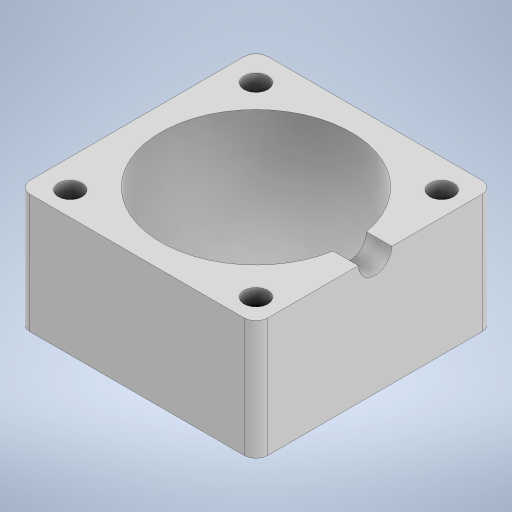
# Autodesk Inventor part: molde1-01
Saved by Autodesk Inventor 2023.2 (Build 272271030, 271C)
## iProperties
Created: 2023-07-19
Part Number: molde1-01
Material: Generic
Document SubType Name: Modeling
Designer: Cris Pat
Density: 1 g/cm^3
Appearance: Default
Author: Cris Pat
Autodesk Inventor part; units mm, degrees
ref_plane "YZ Plane" through (0, 0, 0) normal (1, 0, 0) x (0, 1, 0)
ref_plane "XZ Plane" through (0, 0, 0) normal (0, 1, 0) x (-1, 0, 0)
ref_plane "XY Plane" through (0, 0, 0) normal (0, 0, 1) x (1, 0, 0)
sketch "Sketch1" plane through (0, 0, 0) normal (0, 1, 0) x (-1, 0, 0)
  line L0 (50, 50) -> (-50, 50)
  line L1 (-50, 50) -> (-50, -50)
  line L2 (-50, -50) -> (50, -50)
  line L3 (50, -50) -> (50, 50)
  point P0 (0, 0)
  point P1 (50, 0)
  point P2 (0, 50)
  dimension "d0" = 100
  dimension "d1" = 100
  constraints: 8 end point, 2 midpoint, 2 parallel, 1 horizontal, 1 horizontal alignment, 1 perpendicular, 1 vertical alignment
  measures "d0" distance between parallel lines of L1 L3
  measures "d1" distance between parallel lines of L2 L0
extrude "Extrusion1" add sketch "Sketch1" along normal blind 50
sketch "Sketch2" plane through (0, 50, 0) normal (0, 1, 0) x (1, 0, 0)
  line L0 (50, -50) -> (50, 50) construction
  line L1 (50, 50) -> (-50, 50) construction
  line L2 (-50, 50) -> (-50, -50) construction
  line L3 (-50, -50) -> (50, -50) construction
  line L4 (-50, 50) -> (-50, -50) construction
  line L5 (-50, 0) -> (50, 0) construction
  line L6 (50, -50) -> (50, 50) construction
  arc A0 (40, 0) -> (-40, 0) centre (0, 0) ccw
  line L7 (-40, 0) -> (40, 0) construction
  line L8 (-40, 0) -> (40, 0)
  dimension "d4" = 80
  constraints: 6 end point, 2 collinear, 2 midpoint, 2 point on circle, 2 point on line, 1 centre point, 1 coincident
  measures "d4" diameter of A0
revolve "Revolution1" cut sketch "Sketch2" angle 360 about axis through (-50, 50, 0) along (1, 0, 0)
sketch "Sketch3" plane through (0, 50, 0) normal (0, 1, 0) x (1, 0, 0)
  circle A0 centre (0, 0) radius 40 construction
  line L0 (50, -50) -> (50, 50) construction
  line L1 (50, 50) -> (-50, 50) construction
  line L2 (-50, 50) -> (-50, -50) construction
  line L3 (-50, -50) -> (50, -50) construction
  circle A1 centre (-38, 38) radius 5
  line L4 (50, 50) -> (-50, 50) construction
  line L5 (0, 50) -> (0, 0) construction
  line L6 (0, 0) -> (50, 0) construction
  line L7 (50, -50) -> (50, 50) construction
  dimension "d6" = 10
  dimension "d7" = 12
  dimension "d8" = 12
  constraints: 4 end point, 2 midpoint, 1 centre point, 1 vertical
  measures "d6" diameter of A1
  measures "d7" distance from line of L1 A1.centre
  measures "d8" distance from line of L2 A1.centre
extrude "Extrusion2" cut sketch "Sketch3" against normal blind 50
pattern_linear "Rectangular Pattern1" count 2 spacing 78 along (1, 0, 0) count 2 spacing 78 along (0, 0, 1) of "Extrusion2"
sketch "Sketch4" plane through (50, 0, 50) normal (1, 0, 0) x (0, 0, -1)
  line L0 (0, 0) -> (100, 0) construction
  line L1 (100, 0) -> (100, 50) construction
  line L2 (0, 50) -> (100, 50) construction
  line L3 (0, 0) -> (0, 50) construction
  arc A0 (43, 50) -> (57, 50) centre (50, 50) ccw
  line L4 (57, 50) -> (43, 50)
  line L5 (0, 50) -> (100, 50) projected
  point P0 (50, 0)
  dimension "d17" = 7
  constraints: 2 end point, 2 point on circle, 2 point on line, 1 centre point, 1 coincident, 1 collinear, 1 midpoint
  measures "d17" radius of A0
extrude "Extrusion3" cut sketch "Sketch4" against normal up to surface
fillet "Fillet1" radius 5 4 edges at (-50, 25, 50) (50, 25, 50) (50, 25, -50) (-50, 25, -50)
body "Solid1"
